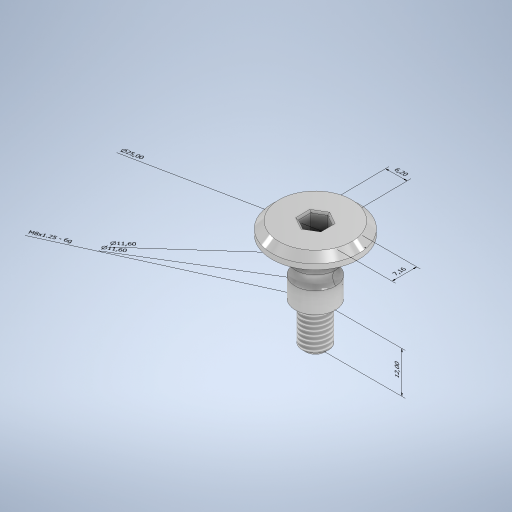
# Autodesk Inventor part: Spindle_Screw
Saved by Autodesk Inventor 2024 (Build 280153000, 153)
## iProperties
Created: 2023-09-23
Part Number: Spindle_Screw
Material: 常规
Document SubType Name: Modeling
Designer: nicx5
Density: 1 g/cm^3
Appearance: 铝 - 黑色
Author: nicx5
Autodesk Inventor part; units mm, degrees
sketch "草图1" plane through (0, 0, 0) normal (0, 1, 0) x (-1, 0, 0)
  circle A0 centre (0, 0) radius 12.5
  circle A1 centre (0, 0) radius 5.8
  dimension "d0" = 25
  dimension "d1" = 11.6
  constraints: 2 centre point
  measures "d0" diameter of A0
  measures "d1" diameter of A1
extrude "拉伸1" add sketch "草图1" along normal blind 3.5 contours A0 | A1
extrude "拉伸2" add sketch "草图1" against normal blind 6 contours A1
ref_plane "工作平面2" through (0, -8, 0) normal (0, -1, 0) x (1, 0, 0)
sketch "草图3" plane through (0, -8, 0) normal (0, -1, 0) x (1, 0, 0)
  circle A0 centre (0, 0) radius 5
  dimension "d10" = 10
  constraints: 1 centre point
  measures "d10" diameter of A0
ref_plane "工作平面1" through (0, -10, 0) normal (0, -1, 0) x (1, 0, 0)
sketch "草图2" plane through (0, -10, 0) normal (0, -1, 0) x (1, 0, 0)
  circle A0 centre (0, 0) radius 5.8 projected
extrude "拉伸3" add sketch "草图2" along normal blind 6
loft "放样1" add profiles "草图3" section 1 edges at (5.8, -6, 0) section 3 edges at (-5.8, -10, 0)
ref_plane "工作平面3" through (0, -16, 0) normal (0, -1, 0) x (1, 0, 0)
sketch "草图4" plane through (0, -16, 0) normal (0, -1, 0) x (1, 0, 0)
  circle A0 centre (0, 0) radius 3.8
  dimension "d18" = 7.6
  constraints: 1 centre point
  measures "d18" diameter of A0
extrude "拉伸4" add sketch "草图4" along normal blind 12
chamfer "倒角1" distance 1 angle 45 1 edges at (-3.8, -28, 0)
chamfer "倒角2" distance 2 angle 45 1 edges at (12.5, 3.5, 0)
sketch "草图5" plane through (0, 3.5, 0) normal (0, 1, 0) x (1, 0, 0)
  circle A0 centre (0, 0) radius 3.1
  line L0 (-3.0786, -1.8264) -> (-3.121, 1.7529)
  line L1 (-3.121, 1.7529) -> (-0.0425, 3.5793)
  line L2 (-0.0425, 3.5793) -> (3.0786, 1.8264)
  line L3 (3.0786, 1.8264) -> (3.121, -1.7529)
  line L4 (3.121, -1.7529) -> (0.0425, -3.5793)
  line L5 (0.0425, -3.5793) -> (-3.0786, -1.8264)
  dimension "d29" = 6.2
  constraints: 12 end point, 1 centre point, 13 other
  measures "d29" diameter of A0
extrude "拉伸5" cut sketch "草图5" against normal blind 5
chamfer "倒角3" distance 0.5 angle 45 6 edges at (3.0998, 3.5, -0.0368) (1.5181, 3.5, -2.7029) (-1.5817, 3.5, -2.6661) (-3.0998, 3.5, 0.0368) (-1.5181, 3.5, 2.7029) (1.5817, 3.5, 2.6661)
thread "螺纹2" size "M8x1.25" class "6g" standard "ISO Metric profile" length 11
